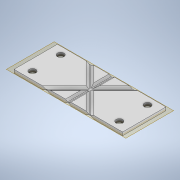
# Autodesk Inventor part: test_hangle_org_2
Saved by Autodesk Inventor 2020 (Build 240168000, 168)
## iProperties
Created: 2021-04-08
Part Number: test_hangle_org_2
Material: Generic
Document SubType Name: Modeling
Designer: Shuang Peng
Density: 1 g/cm^3
Appearance: Default
Author: Shuang Peng
Autodesk Inventor part; units mm, degrees
ref_plane "YZ Plane" through (0, 0, 0) normal (1, 0, 0) x (0, 1, 0)
ref_plane "XZ Plane" through (0, 0, 0) normal (0, 1, 0) x (-1, 0, 0)
ref_plane "XY Plane" through (0, 0, 0) normal (0, 0, 1) x (1, 0, 0)
sketch "Sketch1" plane through (0, 0, 0) normal (0, 1, 0) x (-1, 0, 0)
  line L0 (0, 0) -> (50, 0)
  line L1 (50, 0) -> (50, -20)
  line L2 (50, -20) -> (0, -20)
  line L3 (0, -20) -> (0, 0)
  line L4 (25, 0) -> (25, -20)
  line L5 (25, -20) -> (35, -20)
  line L6 (25, 0) -> (35, 0)
  line L7 (25, 0) -> (15, 0)
  line L8 (25, -20) -> (15, -20)
  line L9 (15, -20) -> (25, -10)
  line L10 (25, -10) -> (15, 0)
  line L11 (25, -10) -> (35, -20)
  line L12 (25, -10) -> (35, 0)
  line L13 (25.25, 2.5) -> (24.75, 2.5)
  line L14 (24.75, 2.5) -> (24.75, -22.5)
  line L15 (24.75, -22.5) -> (25.25, -22.5)
  line L16 (25.25, -22.5) -> (25.25, 2.5)
  line L17 (25.25, 2.5) -> (24.75, -22.5) construction
  line L18 (24.75, 2.5) -> (25.25, -22.5) construction
  line L19 (7.4991, 7.8544) -> (7.1456, 7.5009)
  line L20 (7.1456, 7.5009) -> (42.5009, -27.8544)
  line L21 (42.5009, -27.8544) -> (42.8544, -27.5009)
  line L22 (42.8544, -27.5009) -> (7.4991, 7.8544)
  line L23 (7.4991, 7.8544) -> (42.5009, -27.8544) construction
  line L24 (7.1456, 7.5009) -> (42.8544, -27.5009) construction
  line L25 (42.8544, 7.5009) -> (42.5009, 7.8544)
  line L26 (42.5009, 7.8544) -> (7.1456, -27.5009)
  line L27 (7.1456, -27.5009) -> (7.4991, -27.8544)
  line L28 (7.4991, -27.8544) -> (42.8544, 7.5009)
  line L29 (42.8544, 7.5009) -> (7.1456, -27.5009) construction
  line L30 (42.5009, 7.8544) -> (7.4991, -27.8544) construction
  point P0 (14.6464, -20)
  point P1 (24.6464, -10)
  point P2 (14.6464, 0)
  point P3 (24.75, -10.6036)
  point P4 (15.3536, -20)
  point P5 (24.75, -20)
  point P6 (34.6464, -20)
  point P7 (25.25, -10.6036)
  point P8 (25.25, -20)
  point P9 (15.3536, 0)
  point P10 (24.75, -9.3964)
  point P11 (24.75, 0)
  point P12 (25.25, -9.3964)
  point P13 (34.6464, 0)
  point P14 (25.25, 0)
  point P15 (35.3536, 0)
  point P16 (25.3536, -10)
  point P17 (35.3536, -20)
  dimension "d0" = 50
  dimension "d1" = 20
  dimension "d2" = 10
  dimension "d3" = 10
  dimension "d4" = 10
  dimension "d5" = 10
  dimension "d6" = 0.5
  dimension "d7" = 25
  dimension "d8" = 0.5
  dimension "d9" = 50
  dimension "d10" = 0.5
  dimension "d11" = 50
  constraints: 62 end point, 9 midpoint, 8 parallel, 6 perpendicular, 4 point on line, 2 horizontal
  measures "d0" distance of L1.end L2.end
  measures "d1" distance of L0.end L1.end
  measures "d2" distance of L4.end L5.end
  measures "d3" distance of L4.start L6.end
  measures "d4" distance of L4.start L7.end
  measures "d5" distance of L4.end L8.end
  measures "d6" distance of L13.start L13.end
  measures "d7" distance of L14.end L13.end
  measures "d8" distance of L19.start L19.end
  measures "d9" distance of L20.end L19.end
  measures "d10" distance of L25.start L25.end
  measures "d11" distance of L26.end L25.end
extrude "Extrusion1" add sketch "Sketch1" along normal blind 1.5 contours L0 L20 L26 L2 L3 | L0 L14 L22 | L28 L14 L2 | L0 L26 L16 | L20 L2 L16 | L28 L0 L1 L2 L22
ref_plane "Work Plane1" through (0, 0.75, 0) normal (0, 1, 0) x (1, 0, 0)
sketch "Sketch2" plane through (0, 0.75, 0) normal (0, 1, 0) x (1, 0, 0)
  line L0 (-50, 20) -> (-50, 0) projected
  line L1 (-35.3536, 20) -> (-50, 20) projected
  line L2 (-25.3536, 10) -> (-35.3536, 20) projected
  line L3 (-35.3536, 0) -> (-25.3536, 10) projected
  line L4 (-50, 0) -> (-35.3536, 0) projected
  line L5 (-25.25, 9.3964) -> (-34.6464, 0) projected
  line L6 (-25.25, 0) -> (-25.25, 9.3964) projected
  line L7 (-34.6464, 0) -> (-25.25, 0) projected
  line L8 (-24.75, 9.3964) -> (-24.75, 0) projected
  line L9 (-15.3536, 0) -> (-24.75, 9.3964) projected
  line L10 (-24.75, 0) -> (-15.3536, 0) projected
  line L11 (-24.6464, 10) -> (-14.6464, 0) projected
  line L12 (-14.6464, 20) -> (-24.6464, 10) projected
  line L13 (0, 20) -> (-14.6464, 20) projected
  line L14 (0, 0) -> (0, 20) projected
  line L15 (-14.6464, 0) -> (0, 0) projected
  line L16 (-15.3536, 20) -> (-24.75, 20) projected
  line L17 (-24.75, 10.6036) -> (-15.3536, 20) projected
  line L18 (-24.75, 20) -> (-24.75, 10.6036) projected
  line L19 (-25.25, 20) -> (-34.6464, 20) projected
  line L20 (-25.25, 10.6036) -> (-25.25, 20) projected
  line L21 (-34.6464, 20) -> (-25.25, 10.6036) projected
  line L22 (-50, 0) -> (-35.3536, 0) projected
  line L23 (-50, 0) -> (0, 0)
  line L24 (-50, 20) -> (0, 20)
  constraints: 4 end point, 1 collinear, 1 parallel
extrude "Extrusion2" add sketch "Sketch2" along normal mid plane 0.29 contours L24 L21 L20 L18 L17 L12 L11 L23 L9 L8 L6 L5 L3 L2
chamfer "Chamfer1" distance 1 distance2 0.605 1 edges at (-30.3536, 1.5, -5) measured on face at (-40.2357, 1.5, -13.3333)
chamfer "Chamfer2" distance 1 distance2 0.605 1 edges at (-29.9482, 1.5, -4.6982) measured on face at (-28.3821, 1.5, -3.1321)
chamfer "Chamfer3" distance 1 distance2 0.605 1 edges at (-30.7069, 1.5, -15.3534) measured on face at (-40.7069, 1.5, -13.3333)
chamfer "Chamfer4" distance 1 distance2 0.605 1 edges at (-29.9482, 1.5, -15.3018) measured on face at (-28.3821, 1.5, -16.8679)
chamfer "Chamfer5" distance 1 distance2 0.605 1 edges at (-25.25, 1.5, -16.0085) measured on face at (-27.911, 1.5, -17.339)
chamfer "Chamfer6" distance 1 distance2 0.605 1 edges at (-24.75, 1.5, -15.3018) measured on face at (-21.6179, 1.5, -16.8679)
chamfer "Chamfer7" distance 1 distance2 0.605 1 edges at (-25.25, 1.5, -3.9915) measured on face at (-27.911, 1.5, -2.661)
chamfer "Chamfer8" distance 1 distance2 0.605 1 edges at (-24.75, 1.5, -4.6982) measured on face at (-21.6179, 1.5, -3.1321)
chamfer "Chamfer9" distance 1 distance2 0.605 1 edges at (-19.552, 1.5, -4.1985) measured on face at (-20.9515, 1.5, -2.799)
chamfer "Chamfer10" distance 1 distance2 0.605 1 edges at (-19.6464, 1.5, -5) measured on face at (-9.7643, 1.5, -6.6667)
chamfer "Chamfer11" distance 1 distance2 0.605 1 edges at (-19.552, 1.5, -15.8015) measured on face at (-20.9515, 1.5, -17.201)
chamfer "Chamfer12" distance 1 distance2 0.605 1 edges at (-19.2931, 1.5, -15.3534) measured on face at (-9.2931, 1.5, -13.3333)
chamfer "Chamfer13" distance 0.605 distance2 1 1 edges at (-29.9482, 0, -15.3018) measured on face at (-31.5143, 0.2017, -16.8679)
chamfer "Chamfer14" distance 0.605 distance2 1 1 edges at (-30.3536, 0, -15) measured on face at (-28.6869, 0.2017, -13.3333)
chamfer "Chamfer15" distance 0.605 distance2 1 1 edges at (-25.25, 0, -16.0085) measured on face at (-25.25, 0.4033, -14.2069)
chamfer "Chamfer16" distance 0.605 distance2 1 1 edges at (-24.75, 0, -15.3018) measured on face at (-24.75, 0.2017, -16.8679)
chamfer "Chamfer17" distance 0.605 distance2 1 1 edges at (-19.552, 0, -15.8015) measured on face at (-21.2847, 0.4033, -14.0689)
chamfer "Chamfer18" distance 0.605 distance2 1 1 edges at (-19.6464, 0, -15) measured on face at (-17.9798, 0.2017, -16.6667)
chamfer "Chamfer19" distance 0.605 distance2 1 1 edges at (-19.2931, 0, -4.6466) measured on face at (-21.0775, 0.4033, -6.4311)
chamfer "Chamfer20" distance 0.605 distance2 1 1 edges at (-20.0518, 0, -4.6982) measured on face at (-18.4857, 0.2017, -3.1321)
chamfer "Chamfer21" distance 0.605 distance2 1 1 edges at (-24.75, 0, -3.9915) measured on face at (-24.75, 0.4033, -5.7931)
chamfer "Chamfer22" distance 0.605 distance2 1 1 edges at (-25.25, 0, -4.6982) measured on face at (-25.25, 0.2017, -3.1321)
chamfer "Chamfer23" distance 0.605 distance2 1 1 edges at (-30.448, 0, -4.1985) measured on face at (-28.7153, 0.4033, -5.9311)
chamfer "Chamfer24" distance 0.605 distance2 1 1 edges at (-30.7069, 0, -4.6466) measured on face at (-28.9225, 0.4033, -6.4311)
sketch "Sketch3" plane through (0, 1.5, 0) normal (0, 1, 0) x (1, 0, 0)
  line L0 (-36.7678, 20) -> (-26.7678, 10) projected
  line L1 (-36.7678, 20) -> (-50, 20) projected
  line L2 (-50, 20) -> (-50, 0) projected
  line L3 (-50, 0) -> (-36.7678, 0) projected
  line L4 (-26.7678, 10) -> (-36.7678, 0) projected
  line L5 (-23.2322, 10) -> (-13.2322, 20) projected
  line L6 (-13.2322, 0) -> (-23.2322, 10) projected
  line L7 (-13.2322, 0) -> (0, 0) projected
  line L8 (0, 0) -> (0, 20) projected
  line L9 (0, 20) -> (-13.2322, 20) projected
  line L10 (-26.7678, 10) -> (-23.2322, 10)
  line L11 (-45, 16.5) -> (-45, 3.5)
  line L12 (-45, 3.5) -> (-5, 3.5)
  line L13 (-5, 3.5) -> (-5, 16.5)
  line L14 (-5, 16.5) -> (-45, 16.5)
  line L15 (-45, 16.5) -> (-5, 3.5) construction
  line L16 (-45, 3.5) -> (-5, 16.5) construction
  line L17 (-50, 0) -> (-36.7678, 0) projected
  circle A0 centre (-45, 16.5) radius 1.5
  circle A1 centre (-45, 3.5) radius 1.5
  circle A2 centre (-5, 16.5) radius 1.5
  circle A3 centre (-5, 3.5) radius 1.5
  point P0 (-25, 10)
  dimension "d88" = 13
  dimension "d89" = 40
  dimension "d90" = 3
  dimension "d91" = 3
  dimension "d92" = 3
  dimension "d93" = 3
  constraints: 14 end point, 4 centre point, 4 coincident, 3 midpoint, 2 parallel, 2 perpendicular, 1 horizontal
  measures "d88" distance of L11.start L11.end
  measures "d89" distance of L12.end L11.end
  measures "d90" diameter of A0
  measures "d91" diameter of A1
  measures "d92" diameter of A2
  measures "d93" diameter of A3
extrude "Extrusion3" cut sketch "Sketch3" against normal blind 4 contours A0 L11 L14 | L14 L11 A0 | A2 L13 L14 | L14 L13 A2 | A1 L11 L12 | L12 L11 A1 | A3 L13 L12 | L12 L13 A3
body "Solid1"
